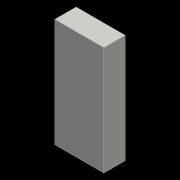
# Autodesk Inventor part: STP_SP
Saved by Autodesk Inventor 2016 (Build 200138000, 138)
## iProperties
Created: 2017-08-22
Part Number: STP_SP
Material: Generic
Document SubType Name: Modeling
Designer: ludwi
Density: 1 g/cm^3
Appearance: Default
Author: ludwi
Autodesk Inventor part; units mm, degrees
ref_plane "YZ Plane" through (0, 0, 0) normal (1, 0, 0) x (0, 1, 0)
ref_plane "XZ Plane" through (0, 0, 0) normal (0, 1, 0) x (-1, 0, 0)
ref_plane "XY Plane" through (0, 0, 0) normal (0, 0, 1) x (1, 0, 0)
sketch "Sketch1" plane through (0, 0, 0) normal (0, 1, 0) x (-1, 0, 0)
  line L0 (57.5, 127.5) -> (-57.5, 127.5)
  line L1 (-57.5, 127.5) -> (-57.5, -127.5)
  line L2 (-57.5, -127.5) -> (57.5, -127.5)
  line L3 (57.5, -127.5) -> (57.5, 127.5)
  point P0 (0, 0)
  point P1 (57.5, 0)
  point P2 (0, -127.5)
  dimension "d0" = 115
  dimension "d1" = 255
  constraints: 8 end point, 2 midpoint, 2 parallel, 1 horizontal, 1 horizontal alignment, 1 perpendicular, 1 vertical alignment
  measures "d0" distance of L1.end L2.end
  measures "d1" distance of L2.end L0.start
extrude "Extrusion1" add sketch "Sketch1" along normal blind 50
body "Solid1"
